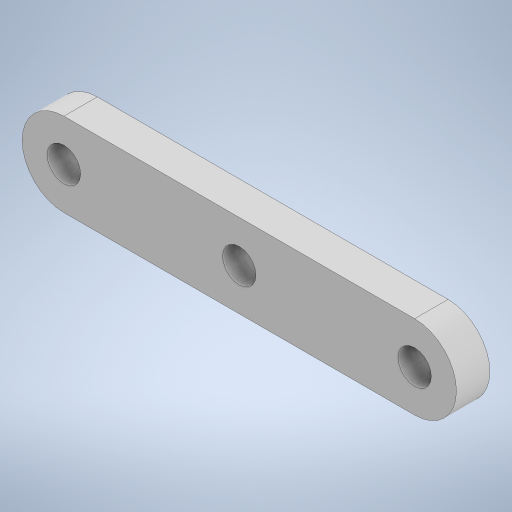
# Autodesk Inventor part: ramię
Saved by Autodesk Inventor 2024 (Build 280153000, 153)
## iProperties
Created: 2024-09-19
Part Number: ramię
Material: Ogólny
Document SubType Name: Modeling
Designer: JEDEN
Density: 1 g/cm^3
Appearance: Domyślna
Author: JEDEN
Autodesk Inventor part; units mm, degrees
ref_plane "YZ Plane" through (0, 0, 0) normal (1, 0, 0) x (0, 1, 0)
ref_plane "XZ Plane" through (0, 0, 0) normal (0, 1, 0) x (-1, 0, 0)
ref_plane "XY Plane" through (0, 0, 0) normal (0, 0, 1) x (1, 0, 0)
sketch "Szkic1" plane through (0, 0, 0) normal (0, 0, 1) x (1, 0, 0)
  line L0 (-25.0296, 0.3305) -> (184.9704, 0.3305) construction
  line L1 (-25.0296, -24.6695) -> (184.9704, -24.6695)
  line L2 (184.9704, 25.3305) -> (-25.0296, 25.3305)
  arc A0 (-25.0296, 25.3305) -> (-25.0296, -24.6695) centre (-25.0296, 0.3305) ccw
  arc A1 (184.9704, -24.6695) -> (184.9704, 25.3305) centre (184.9704, 0.3305) ccw
  circle A2 centre (-25.0296, 0.3305) radius 10
  circle A3 centre (79.9704, 0.3305) radius 10
  circle A4 centre (184.9704, 0.3305) radius 10
  point P0 (0, 0)
  dimension "d0" = 210
  dimension "d1" = 50
  dimension "d2" = 20
  dimension "d3" = 20
  dimension "d4" = 20
  constraints: 8 end point, 5 centre point, 4 point on circle, 4 tangent, 3 coincident, 1 horizontal, 1 midpoint, 1 parallel
  measures "d0" distance of L0.start L0.end
  measures "d1" diameter of A1
  measures "d2" diameter of A2
  measures "d3" diameter of A3
  measures "d4" diameter of A4
extrude "Wyciągnięcie proste1" add sketch "Szkic1" along normal blind 20
